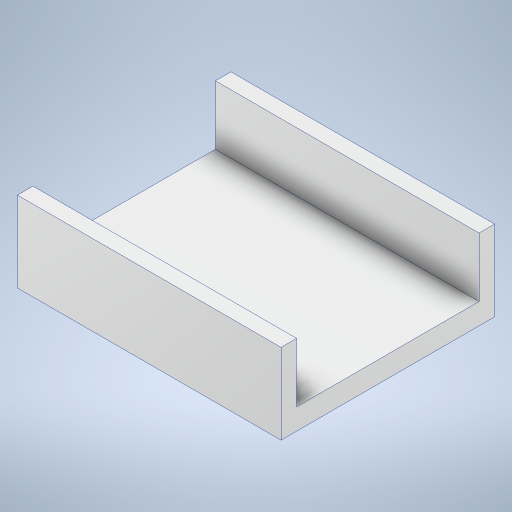
# Autodesk Inventor part: Y_karetka
Saved by Autodesk Inventor 2024 (Build 280153000, 153)
## iProperties
Created: 2023-08-21
Part Number: Y_karetka
Material: Aluminum 6061
Document SubType Name: Modeling
Designer: KirikDK
Mass: 1529.39 g
Surface Area: 1104.64 cm^2
Volume: 566.44 cm^3
Density: 2.7 g/cm^3
Appearance: Aluminum - Flat
Author: KirikDK
Autodesk Inventor part; units mm, degrees
ref_plane "YZ Plane" through (0, 0, 0) normal (1, 0, 0) x (0, 1, 0)
ref_plane "XZ Plane" through (0, 0, 0) normal (0, 1, 0) x (-1, 0, 0)
ref_plane "XY Plane" through (0, 0, 0) normal (0, 0, 1) x (1, 0, 0)
sketch "Sketch1" plane through (0, 0, 0) normal (0, 1, 0) x (-1, 0, 0)
  line L0 (13.84, 69.2) -> (-186.16, 69.2)
  line L1 (-186.16, 69.2) -> (-186.16, -69.2)
  line L2 (-186.16, -69.2) -> (13.84, -69.2)
  line L3 (13.84, -69.2) -> (13.84, 69.2)
  point P0 (0, 0)
  dimension "d0" = 138.4
  dimension "d1" = 200
  constraints: 8 end point, 2 parallel, 1 horizontal, 1 perpendicular
  measures "d0" distance of L2.end L0.start
  measures "d1" distance of L1.end L2.end
extrude "Extrusion1" add sketch "Sketch1" along normal blind 11
sketch "Sketch2" plane through (186.16, 0, 69.2) normal (1, 0, 0) x (0, 0, -1)
  line L0 (0, 0) -> (0, 11) projected
  line L1 (0, 0) -> (-11.8, 0)
  line L2 (-11.8, 0) -> (-11.8, 56)
  line L3 (-11.8, 56) -> (0, 56)
  line L4 (0, 56) -> (0, 0)
  line L5 (138.4, 0) -> (138.4, 11) projected
  line L6 (138.4, 0) -> (150.2, 0)
  line L7 (150.2, 0) -> (150.2, 56)
  line L8 (150.2, 56) -> (138.4, 56)
  line L9 (138.4, 56) -> (138.4, 0)
  point P0 (69.2, 0)
  dimension "d4" = 56
  dimension "d5" = 56
  dimension "d6" = 11.8
  constraints: 16 end point, 5 equal length, 2 horizontal, 2 perpendicular, 1 collinear
  measures "d4" distance between parallel lines of L1 L3
  measures "d5" distance between parallel lines of L6 L8
  measures "d6" distance of L2.end L3.end
extrude "Extrusion2" add sketch "Sketch2" against normal up to surface (200 mm away)
sketch "Sketch3" plane through (0, 0, 0) normal (0, -1, 0) x (1, 0, 0)
  line L0 (186.16, 81) -> (186.16, -81) projected
  line L1 (186.16, 81) -> (-13.84, 81) projected
  line L2 (-13.84, -81) -> (-13.84, 81) projected
  line L3 (186.16, -81) -> (-13.84, -81) projected
  point P0 (0, 0)
extrude "Extrusion3" add sketch "Sketch3" along normal blind 5
body "Solid1"
